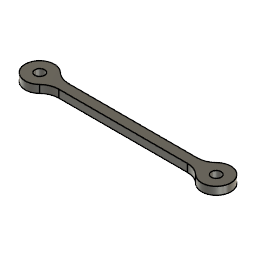
sistem (Autodesk Fusion 360 archive; units mm, degrees)
design "bara"
part number: 2026-04-06-19-36-41-566
Autodesk Fusion 360 part; units mm, degrees
sketch "Sketch1" plane through (0, 0, 0) normal (0, 0, 1) x (1, 0, 0)
  circle A0 centre (0, 0) radius 2.5
  circle A1 centre (0, 0) radius 7.5
  line L0 (0, 2.5) -> (90, 2.5)
  line L1 (0, -2.5) -> (90, -2.5)
  circle A2 centre (90.4068, 0) radius 2.5
  circle A3 centre (90.4068, 0) radius 7.5
  dimension "d1" = 5
  dimension "d2" = 15
  dimension "d3" = 90
  dimension "d4" = 90
  dimension "d5" = 5
  dimension "d6" = 90.4068
  dimension "d7" = 15
  constraint coincident A0.centre A1.centre
  constraint concentric A0 A1
  constraint coincident A0 L0.start
  constraint horizontal L0
  constraint tangent A0 L0
  constraint coincident A0 L1.start
  constraint parallel L0 L1
  constraint tangent A0 L1
  constraint tangent L0 A2
  constraint concentric A2 A3
  measures "d1" diameter of A0
  measures "d2" diameter of A1
  measures "d3" distance of L0.start L0.end
  measures "d4" distance of L1.start L1.end
  measures "d5" diameter of A2
  measures "d6" distance of A0.centre A2.centre
  measures "d7" diameter of A3
extrude "Extrude1" add sketch "Sketch1" along normal blind 4 contours A0 A1 L0 L1 | A0 A1 L0 L1 | A1 L0 L1 A3 | A3
fillet "Fillet1" radius 10 4 edges at (83.3358, 2.5, 2) (7.0711, 2.5, 2) (7.0711, -2.5, 2) (83.3358, -2.5, 2)

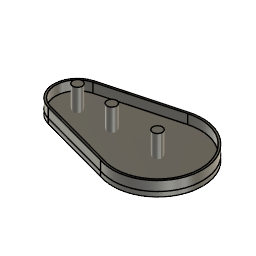
design "suport"
part number: 2026-04-06-19-07-36-977
Autodesk Fusion 360 part; units mm, degrees
sketch "Sketch1" plane through (0, 0, 0) normal (0, 0, 1) x (1, 0, 0)
  circle A0 centre (0, 0) radius 36 construction
  circle A1 centre (0, 0) radius 5
  circle A2 centre (-48, 0) radius 12 construction
  circle A3 centre (-48, 0) radius 24 construction
  circle A4 centre (-48, 0) radius 5
  circle A5 centre (-84, 0) radius 12 construction
  circle A6 centre (-84, 0) radius 5
  line L0 (-90.0238, 22.1972) -> (-11.7857, 43.4292)
  line L1 (-89.9929, -22.2055) -> (-14.772, -42.5063)
  arc A7 (-90.0238, 22.1972) -> (-89.9929, -22.2055) centre (-84, 0) ccw
  arc A8 (-14.772, -42.5063) -> (-11.7857, 43.4292) centre (0, 0) ccw
  arc A9 (-15.3609, -44.419) -> (-12.3095, 45.3594) centre (0, 0) ccw
  line L2 (-90.5476, 24.1273) -> (-12.3095, 45.3594)
  arc A10 (-90.5476, 24.1273) -> (-90.514, -24.1364) centre (-84, 0) ccw
  line L3 (-90.514, -24.1364) -> (-15.3609, -44.419)
  dimension "d1" = 72
  dimension "d2" = 10
  dimension "d3" = 24
  dimension "d4" = 48
  dimension "d5" = 10
  dimension "d6" = 24
  dimension "d7" = 10
  dimension "d11" = 48
  dimension "d16" = 23
  dimension "d17" = 45
  dimension "d18" = -2
  constraint coincident A0.centre A1.centre
  constraint concentric A0 A1
  constraint concentric A2 A3
  constraint concentric A3 A4
  constraint concentric A5 A6
  constraint coincident L0.end A8
  constraint tangent L0 A7
  constraint tangent L1 A7
  constraint concentric A0 A8
  constraint coincident L0 A8.end
  constraint horizontal A2.centre A0.centre
  constraint horizontal A2.centre A5.centre
  constraint tangent A3 A5
  constraint coincident A5.centre A6.centre
  constraint tangent L0 A8
  measures "d1" diameter of A0
  measures "d2" diameter of A1
  measures "d3" diameter of A2
  measures "d4" diameter of A3
  measures "d5" diameter of A4
  measures "d6" diameter of A5
  measures "d7" diameter of A6
  measures "d11" distance of A0.centre A2.centre
  measures "d16" radius of A7
  measures "d17" radius of A8
extrude "Extrude1" add sketch "Sketch1" along normal blind 5 contours A1 | A4 | A6 | L0 L1 A7 A8 makes body 1
extrude "Extrude2" add sketch "Sketch1" along normal blind 5 separate body contours A1 | A4 | A6 | L0 L1 A7 A8 | A9 L2 A10 L3 makes body 2
extrude "Extrude4" add sketch "Sketch1" along normal blind 15 separate body contours A9 L2 A10 L3 makes body 3
extrude "Extrude5" add sketch "Sketch1" along normal blind 28 separate body contours A1 | A4 | A6 makes body 4 at (-79.0248, -0.4978, 18.6667) makes body 5 at (-43.0248, -0.4978, 18.6667) makes body 6 at (4.9752, -0.4978, 18.6667)

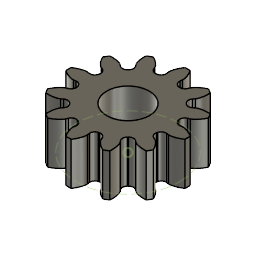
design "rotita1"
part number: 2026-04-06-18-53-35-816
description: Spur Gear; Module: 2.0; Num Teeth: 12; Pressure Angle: 20.0; Backlash: 0.00 mm
part number: 2026-04-06-18-55-15-151
Autodesk Fusion 360 part; units mm, degrees
sketch "Base Circle" plane through (0, 0, 0) normal (0, 0, 1) x (1, 0, 0) in component "Spur Gear 12 teeth"
  circle A0 centre (0, 0) radius 9.686
  circle A1 centre (0, 0) radius 5
extrude "Extrude1" add sketch "Base Circle" along normal blind 10 in component "Spur Gear 12 teeth"
sketch "Gear Tooth" plane through (0, 0, 0) normal (0, 0, 1) x (1, 0, 0) in component "Spur Gear 12 teeth"
  spline S0 degree 5 poles (11.1567, -1.6383) (11.1647, -1.6395) (11.1807, -1.6416) (11.2048, -1.6439) (11.237, -1.6456) (11.2774, -1.6458) (11.318, -1.6445) (11.3587, -1.6423) (11.3994, -1.6396) (11.4401, -1.6366) (11.4809, -1.6333) (11.5218, -1.6295) (11.5626, -1.625) (11.6035, -1.6199) (11.6445, -1.614) (11.6854, -1.6075) (11.7264, -1.6005) (11.7674, -1.5929) (11.8084, -1.585) (11.8494, -1.5766) (11.8905, -1.5678) (11.9315, -1.5587) (11.9725, -1.5491) (12.0135, -1.539) (12.0545, -1.5285) (12.0956, -1.5175) (12.1366, -1.5062) (12.1776, -1.4944) (12.2186, -1.4823) (12.2595, -1.4698) (12.3005, -1.4569) (12.3414, -1.4437) (12.3824, -1.4301) (12.4233, -1.4161) (12.4641, -1.4018) (12.505, -1.3871) (12.5458, -1.372) (12.5866, -1.3566) (12.6274, -1.3409) (12.6681, -1.3248) (12.7088, -1.3084) (12.7495, -1.2917) (12.7902, -1.2746) (12.8308, -1.2572) (12.8713, -1.2395) (12.9119, -1.2215) (12.9523, -1.2031) (12.9928, -1.1844) (13.0332, -1.1654) (13.0735, -1.1461) (13.1138, -1.1265) (13.1541, -1.1066) (13.1943, -1.0863) (13.2345, -1.0658) (13.2746, -1.045) (13.3146, -1.0239) (13.3546, -1.0024) (13.3946, -0.9807) (13.4344, -0.9587) (13.4743, -0.9364) (13.514, -0.9138) (13.5538, -0.8909) (13.5934, -0.8678) (13.633, -0.8443) (13.6725, -0.8206) (13.712, -0.7966) (13.7514, -0.7723) (13.7907, -0.7477) (13.8299, -0.7229) (13.8691, -0.6978) (13.9082, -0.6724) (13.9395, -0.6518) (13.9629, -0.6363) (13.9784, -0.6259) (13.9862, -0.6207) knots 0 0 0 0 0 0 0.01428571 0.02857143 0.04285714 0.05714286 0.07142857 0.08571429 0.1 0.11428571 0.12857143 0.14285714 0.15714286 0.17142857 0.18571429 0.2 0.21428571 0.22857143 0.24285714 0.25714286 0.27142857 0.28571429 0.3 0.31428571 0.32857143 0.34285714 0.35714286 0.37142857 0.38571429 0.4 0.41428571 0.42857143 0.44285714 0.45714286 0.47142857 0.48571429 0.5 0.51428571 0.52857143 0.54285714 0.55714286 0.57142857 0.58571429 0.6 0.61428571 0.62857143 0.64285714 0.65714286 0.67142857 0.68571429 0.7 0.71428571 0.72857143 0.74285714 0.75714286 0.77142857 0.78571429 0.8 0.81428571 0.82857143 0.84285714 0.85714286 0.87142857 0.88571429 0.9 0.91428571 0.92857143 0.94285714 0.95714286 0.97142857 0.98571429 1 1 1 1 1 1
  spline S1 degree 5 poles (11.1567, 1.6383) (11.1647, 1.6395) (11.1807, 1.6416) (11.2048, 1.6439) (11.237, 1.6456) (11.2774, 1.6458) (11.318, 1.6445) (11.3587, 1.6423) (11.3994, 1.6396) (11.4401, 1.6366) (11.4809, 1.6333) (11.5218, 1.6295) (11.5626, 1.625) (11.6035, 1.6199) (11.6445, 1.614) (11.6854, 1.6075) (11.7264, 1.6005) (11.7674, 1.5929) (11.8084, 1.585) (11.8494, 1.5766) (11.8905, 1.5678) (11.9315, 1.5587) (11.9725, 1.5491) (12.0135, 1.539) (12.0545, 1.5285) (12.0956, 1.5175) (12.1366, 1.5062) (12.1776, 1.4944) (12.2186, 1.4823) (12.2595, 1.4698) (12.3005, 1.4569) (12.3414, 1.4437) (12.3824, 1.4301) (12.4233, 1.4161) (12.4641, 1.4018) (12.505, 1.3871) (12.5458, 1.372) (12.5866, 1.3566) (12.6274, 1.3409) (12.6681, 1.3248) (12.7088, 1.3084) (12.7495, 1.2917) (12.7902, 1.2746) (12.8308, 1.2572) (12.8713, 1.2395) (12.9119, 1.2215) (12.9523, 1.2031) (12.9928, 1.1844) (13.0332, 1.1654) (13.0735, 1.1461) (13.1138, 1.1265) (13.1541, 1.1066) (13.1943, 1.0863) (13.2345, 1.0658) (13.2746, 1.045) (13.3146, 1.0239) (13.3546, 1.0024) (13.3946, 0.9807) (13.4344, 0.9587) (13.4743, 0.9364) (13.514, 0.9138) (13.5538, 0.8909) (13.5934, 0.8678) (13.633, 0.8443) (13.6725, 0.8206) (13.712, 0.7966) (13.7514, 0.7723) (13.7907, 0.7477) (13.8299, 0.7229) (13.8691, 0.6978) (13.9082, 0.6724) (13.9395, 0.6518) (13.9629, 0.6363) (13.9784, 0.6259) (13.9862, 0.6207) knots 0 0 0 0 0 0 0.01428571 0.02857143 0.04285714 0.05714286 0.07142857 0.08571429 0.1 0.11428571 0.12857143 0.14285714 0.15714286 0.17142857 0.18571429 0.2 0.21428571 0.22857143 0.24285714 0.25714286 0.27142857 0.28571429 0.3 0.31428571 0.32857143 0.34285714 0.35714286 0.37142857 0.38571429 0.4 0.41428571 0.42857143 0.44285714 0.45714286 0.47142857 0.48571429 0.5 0.51428571 0.52857143 0.54285714 0.55714286 0.57142857 0.58571429 0.6 0.61428571 0.62857143 0.64285714 0.65714286 0.67142857 0.68571429 0.7 0.71428571 0.72857143 0.74285714 0.75714286 0.77142857 0.78571429 0.8 0.81428571 0.82857143 0.84285714 0.85714286 0.87142857 0.88571429 0.9 0.91428571 0.92857143 0.94285714 0.95714286 0.97142857 0.98571429 1 1 1 1 1 1
  arc A0 (13.9862, -0.6207) -> (13.9862, 0.6207) centre (0, 0) ccw
  line L0 (9.5733, -1.4058) -> (11.1567, -1.6383)
  line L1 (9.5733, 1.4058) -> (11.1567, 1.6383)
  line L2 (9.5733, -1.4058) -> (9.5733, 1.4058)
  point P0 (11.3527, -1.6425)
  point P1 (11.5515, -1.6261)
  point P2 (11.7521, -1.5957)
  point P3 (11.954, -1.5533)
  point P4 (12.1568, -1.5003)
  point P5 (12.3603, -1.4374)
  point P6 (12.5642, -1.3651)
  point P7 (12.7683, -1.2838)
  point P8 (12.9724, -1.1938)
  point P9 (13.1764, -1.0953)
  point P10 (13.3799, -0.9887)
  point P11 (13.5828, -0.8739)
  point P12 (13.785, -0.7512)
  point P13 (11.3527, 1.6425)
  point P14 (11.5515, 1.6261)
  point P15 (11.7521, 1.5957)
  point P16 (11.954, 1.5533)
  point P17 (12.1568, 1.5003)
  point P18 (12.3603, 1.4374)
  point P19 (12.5642, 1.3651)
  point P20 (12.7683, 1.2838)
  point P21 (12.9724, 1.1938)
  point P22 (13.1764, 1.0953)
  point P23 (13.3799, 0.9887)
  point P24 (13.5828, 0.8739)
  point P25 (13.785, 0.7512)
extrude "Extrude2" add sketch "Gear Tooth" along normal blind 10 in component "Spur Gear 12 teeth"
fillet "Fillet1" radius 1.15 2 edges at (9.5832, -1.4073, 5) (9.5832, 1.4073, 5) in component "Spur Gear 12 teeth"
pattern_circular "C-Pattern1" count 12 over 360 about axis through (0, 0, 0) along (0, 0, 1) of "Extrude2", "Fillet1" in component "Spur Gear 12 teeth"
sketch "Diametrial Pitch Circle" plane through (0, 0, 0) normal (0, 0, 1) x (1, 0, 0) in component "Spur Gear 12 teeth"
  circle A0 centre (0, 0) radius 12 construction
component "Spur Gear 12 teeth" placed x (1, 0, 0) y (0, 1, 0) z (0, 0, 1) at (0, 0, 0)

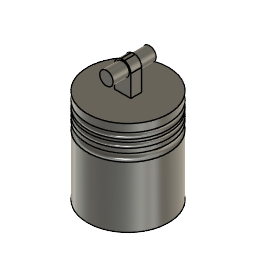
design "piston"
part number: 2026-04-06-19-49-58-247
Autodesk Fusion 360 part; units mm, degrees
sketch "Sketch2" plane through (0, 0, 0) normal (0, 1, 0) x (1, 0, 0)
  line L0 (0, 0) -> (15, 0)
  line L1 (15, -35) -> (0, -35)
  line L2 (0, -35) -> (0, 0)
  line L3 (-3.048, -35) -> (3.048, -35)
  line L4 (3.048, -35) -> (3.048, -43)
  line L5 (0.665, -45.9746) -> (-0.665, -45.9746)
  line L6 (-3.048, -43) -> (-3.048, -35)
  circle A0 centre (0, -43) radius 3.048
  arc A1 (15, -29.936) -> (15, -32.064) centre (15, -31) ccw
  arc A2 (15, -27.0482) -> (15, -28.9518) centre (15, -28) ccw
  arc A3 (15, -22.5858) -> (15, -25.4142) centre (15, -24) ccw
  line L7 (15, -32.064) -> (15, -35)
  line L8 (15, -28.9518) -> (15, -29.936)
  line L9 (15, 0) -> (15, -22.5858)
  line L10 (15, -25.4142) -> (15, -27.0482)
  circle A4 centre (0, -43) radius 2.5
  dimension "d3" = 15
  dimension "d4" = 35
  dimension "d6" = 6.096
  dimension "d7" = 35
  dimension "d8" = 8
  dimension "d10" = 3.048
  dimension "d20" = 5
  constraint horizontal L0
  constraint vertical L9
  constraint horizontal L1
  constraint vertical L2
  constraint coincident L0.start L2.end
  constraint horizontal L3
  constraint vertical L4
  constraint horizontal L5
  constraint vertical L6
  constraint coincident A0 L6.start
  constraint coincident A0 L5.end
  constraint coincident A0 L5.start
  constraint coincident A0 L4.end
  constraint tangent L6 A0
  constraint tangent L4 A0
  constraint coincident A1.centre L8
  constraint coincident A2.centre L10
  constraint coincident A3.centre L9
  constraint collinear L7 L8
  constraint collinear L8 L10
  constraint collinear L9 L10
  constraint concentric A0 A4
  measures "d3" distance of L0.start L0.end
  measures "d4" distance of L0.start L1.end
  measures "d6" distance of L4 L6
  measures "d7" distance of L0 L3
  measures "d8" distance of L3 A0.centre
  measures "d10" distance of L0.start L6
  measures "d20" diameter of A4
extrude "Extrude1" add sketch "Sketch2" along normal blind 2 and the other way blind 2 contours L1 L3 L4 L6 A0 | L5 A0 | A4 picked at (0.0623, -45.814)
revolve "Revolve2" add sketch "Sketch2" angle 360 about axis through (0, 0, 35) along (0, 0, -1) contours L0 L1 L2 L3 A1 A2 A3 L7 L8 L9 L10
extrude "Extrude3" add sketch "Sketch2" along normal blind 8 and the other way blind 8 contours A4

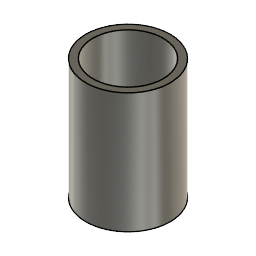
design "cilindru"
part number: 2026-04-06-23-18-16-083
Autodesk Fusion 360 part; units mm, degrees
sketch "Sketch1" plane through (0, 0, 0) normal (0, 0, 1) x (1, 0, 0)
  circle A0 centre (0, 0) radius 17.5
  circle A1 centre (0, 0) radius 21
  dimension "d1" = 35
  dimension "d2" = 42
  constraint coincident A0.centre A1.centre
  constraint concentric A0 A1
  measures "d1" diameter of A0
  measures "d2" diameter of A1
extrude "Extrude1" add sketch "Sketch1" along normal blind 5 contours A0 | A1
extrude "Extrude2" add sketch "Sketch1" along normal blind 60

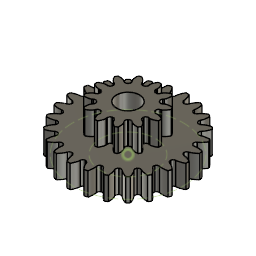
design "rotita2"
part number: 2026-04-06-18-55-30-373
description: Spur Gear; Module: 2.0; Num Teeth: 24; Pressure Angle: 20.0; Backlash: 0.00 mm
part number: 2026-04-06-18-55-53-550
description: Spur Gear; Module: 2.0; Num Teeth: 12; Pressure Angle: 20.0; Backlash: 0.00 mm
part number: 2026-04-06-18-56-12-533
Autodesk Fusion 360 part; units mm, degrees
sketch "Base Circle" plane through (0, 0, 0) normal (0, 0, 1) x (1, 0, 0) in component "Spur Gear 24 teeth"
  circle A0 centre (0, 0) radius 21.686
  circle A1 centre (0, 0) radius 5
extrude "Extrude1" add sketch "Base Circle" along normal blind 10 contours A0 picked at (16.024646, -1.325781) makes body 1 in component "Spur Gear 24 teeth"
sketch "Gear Tooth" plane through (0, 0, 0) normal (0, 0, 1) x (1, 0, 0) in component "Spur Gear 24 teeth"
  spline S0 degree 5 poles (22.479853, -1.810249) (22.489932, -1.811061) (22.510097, -1.812431) (22.540365, -1.813726) (22.580762, -1.814006) (22.631316, -1.812378) (22.681918, -1.80932) (22.732555, -1.805377) (22.783217, -1.800952) (22.833897, -1.796205) (22.88459, -1.791127) (22.935292, -1.785606) (22.986001, -1.7795) (23.036714, -1.772707) (23.087429, -1.765222) (23.138144, -1.757096) (23.188857, -1.748415) (23.239566, -1.739269) (23.290268, -1.729725) (23.340962, -1.719806) (23.391647, -1.70951) (23.442321, -1.698818) (23.492983, -1.687708) (23.543632, -1.676168) (23.594266, -1.664202) (23.644885, -1.651825) (23.695488, -1.639058) (23.746072, -1.62592) (23.796638, -1.612428) (23.847183, -1.598588) (23.897708, -1.584404) (23.94821, -1.569874) (23.99869, -1.554999) (24.049146, -1.539779) (24.099578, -1.524219) (24.149984, -1.508324) (24.200363, -1.4921) (24.250715, -1.475555) (24.30104, -1.458693) (24.351335, -1.441519) (24.401601, -1.424035) (24.451836, -1.406244) (24.50204, -1.388148) (24.552212, -1.369748) (24.602351, -1.351049) (24.652457, -1.332052) (24.702529, -1.312762) (24.752565, -1.293182) (24.802567, -1.273314) (24.852531, -1.25316) (24.902459, -1.232724) (24.952349, -1.212006) (25.0022, -1.19101) (25.052013, -1.169738) (25.101786, -1.14819) (25.151518, -1.126371) (25.201209, -1.104281) (25.250858, -1.081923) (25.300465, -1.059298) (25.350029, -1.036409) (25.399549, -1.013256) (25.449026, -0.989843) (25.498457, -0.96617) (25.547843, -0.942239) (25.597183, -0.918052) (25.646476, -0.893611) (25.695722, -0.868917) (25.744919, -0.843972) (25.794067, -0.818777) (25.843166, -0.793334) (25.892215, -0.767643) (25.931415, -0.746893) (25.960793, -0.73122) (25.980369, -0.720722) (25.990154, -0.71546) knots 0 0 0 0 0 0 0.01428571 0.02857143 0.04285714 0.05714286 0.07142857 0.08571429 0.1 0.11428571 0.12857143 0.14285714 0.15714286 0.17142857 0.18571429 0.2 0.21428571 0.22857143 0.24285714 0.25714286 0.27142857 0.28571429 0.3 0.31428571 0.32857143 0.34285714 0.35714286 0.37142857 0.38571429 0.4 0.41428571 0.42857143 0.44285714 0.45714286 0.47142857 0.48571429 0.5 0.51428571 0.52857143 0.54285714 0.55714286 0.57142857 0.58571429 0.6 0.61428571 0.62857143 0.64285714 0.65714286 0.67142857 0.68571429 0.7 0.71428571 0.72857143 0.74285714 0.75714286 0.77142857 0.78571429 0.8 0.81428571 0.82857143 0.84285714 0.85714286 0.87142857 0.88571429 0.9 0.91428571 0.92857143 0.94285714 0.95714286 0.97142857 0.98571429 1 1 1 1 1 1
  spline S1 degree 5 poles (22.479853, 1.810249) (22.489932, 1.811061) (22.510097, 1.812431) (22.540365, 1.813726) (22.580762, 1.814006) (22.631316, 1.812378) (22.681918, 1.80932) (22.732555, 1.805377) (22.783217, 1.800952) (22.833897, 1.796205) (22.88459, 1.791127) (22.935292, 1.785606) (22.986001, 1.7795) (23.036714, 1.772707) (23.087429, 1.765222) (23.138144, 1.757096) (23.188857, 1.748415) (23.239566, 1.739269) (23.290268, 1.729725) (23.340962, 1.719806) (23.391647, 1.70951) (23.442321, 1.698818) (23.492983, 1.687708) (23.543632, 1.676168) (23.594266, 1.664202) (23.644885, 1.651825) (23.695488, 1.639058) (23.746072, 1.62592) (23.796638, 1.612428) (23.847183, 1.598588) (23.897708, 1.584404) (23.94821, 1.569874) (23.99869, 1.554999) (24.049146, 1.539779) (24.099578, 1.524219) (24.149984, 1.508324) (24.200363, 1.4921) (24.250715, 1.475555) (24.30104, 1.458693) (24.351335, 1.441519) (24.401601, 1.424035) (24.451836, 1.406244) (24.50204, 1.388148) (24.552212, 1.369748) (24.602351, 1.351049) (24.652457, 1.332052) (24.702529, 1.312762) (24.752565, 1.293182) (24.802567, 1.273314) (24.852531, 1.25316) (24.902459, 1.232724) (24.952349, 1.212006) (25.0022, 1.19101) (25.052013, 1.169738) (25.101786, 1.14819) (25.151518, 1.126371) (25.201209, 1.104281) (25.250858, 1.081923) (25.300465, 1.059298) (25.350029, 1.036409) (25.399549, 1.013256) (25.449026, 0.989843) (25.498457, 0.96617) (25.547843, 0.942239) (25.597183, 0.918052) (25.646476, 0.893611) (25.695722, 0.868917) (25.744919, 0.843972) (25.794067, 0.818777) (25.843166, 0.793334) (25.892215, 0.767643) (25.931415, 0.746893) (25.960793, 0.73122) (25.980369, 0.720722) (25.990154, 0.71546) knots 0 0 0 0 0 0 0.01428571 0.02857143 0.04285714 0.05714286 0.07142857 0.08571429 0.1 0.11428571 0.12857143 0.14285714 0.15714286 0.17142857 0.18571429 0.2 0.21428571 0.22857143 0.24285714 0.25714286 0.27142857 0.28571429 0.3 0.31428571 0.32857143 0.34285714 0.35714286 0.37142857 0.38571429 0.4 0.41428571 0.42857143 0.44285714 0.45714286 0.47142857 0.48571429 0.5 0.51428571 0.52857143 0.54285714 0.55714286 0.57142857 0.58571429 0.6 0.61428571 0.62857143 0.64285714 0.65714286 0.67142857 0.68571429 0.7 0.71428571 0.72857143 0.74285714 0.75714286 0.77142857 0.78571429 0.8 0.81428571 0.82857143 0.84285714 0.85714286 0.87142857 0.88571429 0.9 0.91428571 0.92857143 0.94285714 0.95714286 0.97142857 0.98571429 1 1 1 1 1 1
  arc A0 (25.990154, -0.71546) -> (25.990154, 0.71546) centre (0, 0) ccw
  line L0 (21.606059, -1.739885) -> (22.479853, -1.810249)
  line L1 (21.606059, 1.739885) -> (22.479853, 1.810249)
  line L2 (21.606059, -1.739885) -> (21.606059, 1.739885)
  point P0 (22.727246, -1.805688)
  point P1 (22.976216, -1.780562)
  point P2 (23.22614, -1.741628)
  point P3 (23.476751, -1.691207)
  point P4 (23.727867, -1.630599)
  point P5 (23.979338, -1.560655)
  point P6 (24.231035, -1.481979)
  point P7 (24.482841, -1.395027)
  point P8 (24.734647, -1.300153)
  point P9 (24.986349, -1.197645)
  point P10 (25.237847, -1.087738)
  point P11 (25.489043, -0.97063)
  point P12 (25.739844, -0.846489)
  point P13 (22.727246, 1.805688)
  point P14 (22.976216, 1.780562)
  point P15 (23.22614, 1.741628)
  point P16 (23.476751, 1.691207)
  point P17 (23.727867, 1.630599)
  point P18 (23.979338, 1.560655)
  point P19 (24.231035, 1.481979)
  point P20 (24.482841, 1.395027)
  point P21 (24.734647, 1.300153)
  point P22 (24.986349, 1.197645)
  point P23 (25.237847, 1.087738)
  point P24 (25.489043, 0.97063)
  point P25 (25.739844, 0.846489)
extrude "Extrude2" add sketch "Gear Tooth" along normal blind 10 contours S0 S1 A0 L0 L1 L2 picked at (22.188588, -0.579962) bodies 1 in component "Spur Gear 24 teeth"
fillet "Fillet1" radius 1.15 2 edges at (21.616027, -1.740687, 5) (21.616027, 1.740687, 5) on bodies 1 in component "Spur Gear 24 teeth"
pattern_circular "C-Pattern1" count 24 over 360 about axis through (0, 0, 0) along (0, 0, 1) of "Extrude2", "Fillet1" in component "Spur Gear 24 teeth"
sketch "Diametrial Pitch Circle" plane through (0, 0, 0) normal (0, 0, 1) x (1, 0, 0) in component "Spur Gear 24 teeth"
  circle A0 centre (0, 0) radius 24 construction
sketch "Base Circle (2)" plane through (0, 0, 0) normal (0, 0, 1) x (1, 0, 0) in component "Spur Gear 12 teeth"
  circle A0 centre (0, 0) radius 9.686
  circle A1 centre (0, 0) radius 5
extrude "Extrude1'" add sketch "Base Circle (2)" along normal blind 10 separate body contours A0 picked at (8.069323, -0.729612) makes body 2 in component "Spur Gear 12 teeth"
sketch "Gear Tooth (2)" plane through (0, 0, 0) normal (0, 0, 1) x (1, 0, 0) in component "Spur Gear 12 teeth"
  spline S0 degree 5 poles (11.156663, -1.638313) (11.164659, -1.639487) (11.180671, -1.641579) (11.20475, -1.643949) (11.236974, -1.645648) (11.277421, -1.645778) (11.317995, -1.644473) (11.358658, -1.642285) (11.399376, -1.639617) (11.440135, -1.636617) (11.480927, -1.633269) (11.521753, -1.629454) (11.562616, -1.625026) (11.603517, -1.619888) (11.644453, -1.614039) (11.685417, -1.607534) (11.726404, -1.600462) (11.767405, -1.592915) (11.808416, -1.584954) (11.849432, -1.5766) (11.890452, -1.567846) (11.931476, -1.558673) (11.9725, -1.549057) (12.013525, -1.538987) (12.054549, -1.528471) (12.095567, -1.517524) (12.136579, -1.506165) (12.17758, -1.494416) (12.218569, -1.482291) (12.259544, -1.469795) (12.300502, -1.45693) (12.341443, -1.443697) (12.382365, -1.430093) (12.423266, -1.416121) (12.464144, -1.401785) (12.504999, -1.387089) (12.545827, -1.372042) (12.586628, -1.356648) (12.627399, -1.340914) (12.66814, -1.324842) (12.708848, -1.308435) (12.749522, -1.291696) (12.790161, -1.274626) (12.830763, -1.257228) (12.871327, -1.239505) (12.911852, -1.221459) (12.952335, -1.203093) (12.992776, -1.184412) (13.033174, -1.165417) (13.073526, -1.146111) (13.113831, -1.126496) (13.154089, -1.106575) (13.194298, -1.086348) (13.234457, -1.065819) (13.274563, -1.044989) (13.314617, -1.023861) (13.354617, -1.002436) (13.39456, -0.980716) (13.434448, -0.958705) (13.474277, -0.936402) (13.514047, -0.91381) (13.553757, -0.890931) (13.593407, -0.867766) (13.632993, -0.844316) (13.672516, -0.820585) (13.711973, -0.796573) (13.751363, -0.772282) (13.790685, -0.747715) (13.829938, -0.722872) (13.869121, -0.697754) (13.908235, -0.672363) (13.939469, -0.651832) (13.962864, -0.636311) (13.978446, -0.625909) (13.986234, -0.620695) knots 0 0 0 0 0 0 0.01428571 0.02857143 0.04285714 0.05714286 0.07142857 0.08571429 0.1 0.11428571 0.12857143 0.14285714 0.15714286 0.17142857 0.18571429 0.2 0.21428571 0.22857143 0.24285714 0.25714286 0.27142857 0.28571429 0.3 0.31428571 0.32857143 0.34285714 0.35714286 0.37142857 0.38571429 0.4 0.41428571 0.42857143 0.44285714 0.45714286 0.47142857 0.48571429 0.5 0.51428571 0.52857143 0.54285714 0.55714286 0.57142857 0.58571429 0.6 0.61428571 0.62857143 0.64285714 0.65714286 0.67142857 0.68571429 0.7 0.71428571 0.72857143 0.74285714 0.75714286 0.77142857 0.78571429 0.8 0.81428571 0.82857143 0.84285714 0.85714286 0.87142857 0.88571429 0.9 0.91428571 0.92857143 0.94285714 0.95714286 0.97142857 0.98571429 1 1 1 1 1 1
  spline S1 degree 5 poles (11.156663, 1.638313) (11.164659, 1.639487) (11.180671, 1.641579) (11.20475, 1.643949) (11.236974, 1.645648) (11.277421, 1.645778) (11.317995, 1.644473) (11.358658, 1.642285) (11.399376, 1.639617) (11.440135, 1.636617) (11.480927, 1.633269) (11.521753, 1.629454) (11.562616, 1.625026) (11.603517, 1.619888) (11.644453, 1.614039) (11.685417, 1.607534) (11.726404, 1.600462) (11.767405, 1.592915) (11.808416, 1.584954) (11.849432, 1.5766) (11.890452, 1.567846) (11.931476, 1.558673) (11.9725, 1.549057) (12.013525, 1.538987) (12.054549, 1.528471) (12.095567, 1.517524) (12.136579, 1.506165) (12.17758, 1.494416) (12.218569, 1.482291) (12.259544, 1.469795) (12.300502, 1.45693) (12.341443, 1.443697) (12.382365, 1.430093) (12.423266, 1.416121) (12.464144, 1.401785) (12.504999, 1.387089) (12.545827, 1.372042) (12.586628, 1.356648) (12.627399, 1.340914) (12.66814, 1.324842) (12.708848, 1.308435) (12.749522, 1.291696) (12.790161, 1.274626) (12.830763, 1.257228) (12.871327, 1.239505) (12.911852, 1.221459) (12.952335, 1.203093) (12.992776, 1.184412) (13.033174, 1.165417) (13.073526, 1.146111) (13.113831, 1.126496) (13.154089, 1.106575) (13.194298, 1.086348) (13.234457, 1.065819) (13.274563, 1.044989) (13.314617, 1.023861) (13.354617, 1.002436) (13.39456, 0.980716) (13.434448, 0.958705) (13.474277, 0.936402) (13.514047, 0.91381) (13.553757, 0.890931) (13.593407, 0.867766) (13.632993, 0.844316) (13.672516, 0.820585) (13.711973, 0.796573) (13.751363, 0.772282) (13.790685, 0.747715) (13.829938, 0.722872) (13.869121, 0.697754) (13.908235, 0.672363) (13.939469, 0.651832) (13.962864, 0.636311) (13.978446, 0.625909) (13.986234, 0.620695) knots 0 0 0 0 0 0 0.01428571 0.02857143 0.04285714 0.05714286 0.07142857 0.08571429 0.1 0.11428571 0.12857143 0.14285714 0.15714286 0.17142857 0.18571429 0.2 0.21428571 0.22857143 0.24285714 0.25714286 0.27142857 0.28571429 0.3 0.31428571 0.32857143 0.34285714 0.35714286 0.37142857 0.38571429 0.4 0.41428571 0.42857143 0.44285714 0.45714286 0.47142857 0.48571429 0.5 0.51428571 0.52857143 0.54285714 0.55714286 0.57142857 0.58571429 0.6 0.61428571 0.62857143 0.64285714 0.65714286 0.67142857 0.68571429 0.7 0.71428571 0.72857143 0.74285714 0.75714286 0.77142857 0.78571429 0.8 0.81428571 0.82857143 0.84285714 0.85714286 0.87142857 0.88571429 0.9 0.91428571 0.92857143 0.94285714 0.95714286 0.97142857 0.98571429 1 1 1 1 1 1
  arc A0 (13.986234, -0.620695) -> (13.986234, 0.620695) centre (0, 0) ccw
  line L0 (9.573332, -1.405807) -> (11.156663, -1.638313)
  line L1 (9.573332, 1.405807) -> (11.156663, 1.638313)
  line L2 (9.573332, -1.405807) -> (9.573332, 1.405807)
  point P0 (11.352656, -1.642513)
  point P1 (11.551515, -1.626125)
  point P2 (11.752126, -1.59567)
  point P3 (11.954009, -1.553334)
  point P4 (12.156828, -1.500315)
  point P5 (12.360311, -1.437377)
  point P6 (12.564219, -1.365058)
  point P7 (12.768332, -1.283752)
  point P8 (12.972443, -1.193763)
  point P9 (13.176355, -1.095333)
  point P10 (13.379875, -0.988658)
  point P11 (13.582818, -0.873903)
  point P12 (13.784998, -0.751208)
  point P13 (11.352656, 1.642513)
  point P14 (11.551515, 1.626125)
  point P15 (11.752126, 1.59567)
  point P16 (11.954009, 1.553334)
  point P17 (12.156828, 1.500315)
  point P18 (12.360311, 1.437377)
  point P19 (12.564219, 1.365058)
  point P20 (12.768332, 1.283752)
  point P21 (12.972443, 1.193763)
  point P22 (13.176355, 1.095333)
  point P23 (13.379875, 0.988658)
  point P24 (13.582818, 0.873903)
  point P25 (13.784998, 0.751208)
extrude "Extrude2'" add sketch "Gear Tooth (2)" along normal blind 10 contours S0 S1 A0 L0 L1 L2 picked at (10.628886, -0.468602) bodies 2 in component "Spur Gear 12 teeth"
fillet "Fillet1'" radius 1.15 2 edges at (9.583226, -1.40726, 5) (9.583226, 1.40726, 5) on bodies 2 in component "Spur Gear 12 teeth"
pattern_circular "C-Pattern1'" count 12 over 360 about axis through (0, 0, 0) along (0, 0, 1) of "Extrude2'", "Fillet1'" in component "Spur Gear 12 teeth"
sketch "Diametrial Pitch Circle (2)" plane through (0, 0, 0) normal (0, 0, 1) x (1, 0, 0) in component "Spur Gear 12 teeth"
  circle A0 centre (0, 0) radius 12 construction
move_body "Move1" bodies 2 to x (1, 0, 0) y (0, 1, 0) z (0, 0, 1) at (0, 0, 10) in component "Spur Gear 12 teeth"
combine "Combine1" operation add target body 2 tool bodies 1 in component "Spur Gear 12 teeth"
component "Spur Gear 24 teeth" placed x (1, 0, 0) y (0, 1, 0) z (0, 0, 1) at (0, 0, 0)
component "Spur Gear 12 teeth" placed x (1, 0, 0) y (0, 1, 0) z (0, 0, 1) at (0, 0, 0)
